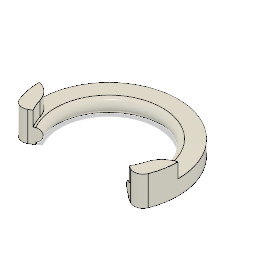
socket_clip (Autodesk Fusion 360 design; units mm, degrees)
Autodesk Fusion 360 part; units mm, degrees
sketch "Sketch6" plane through (0, 0, 0) normal (0, 1, 0) x (1, 0, 0)
  circle A0 centre (0, 0) radius 12
  circle A1 centre (0, 0) radius 9
  dimension "d1" = 24
  dimension "d2" = -3
  constraint coincident A0.centre A1.centre
  measures "d1" diameter of A0
sketch "Sketch3" plane through (0, 0, 0) normal (0, 1, 0) x (1, 0, 0)
  circle A0 centre (0, 0) radius 12.125
  circle A1 centre (0, 0) radius 14.125
  line L0 (0, 0) -> (13.125, 0) construction
  dimension "d18" = 24.25
  dimension "d22" = 2
  constraint coincident A0.centre A1.centre
  constraint horizontal L0
  measures "d18" diameter of A0
sketch "Sketch4" plane through (0, 0, 0) normal (0, 0, 1) x (1, 0, 0)
  line L0 (12.125, 0) -> (10.625, 0)
  line L1 (10.625, 0) -> (10.625, 2.8)
  line L2 (10.625, 2.8) -> (12.125, 2.8)
  line L3 (12.125, 2.8) -> (12.125, 0)
  arc A0 (12.125, 2.8) -> (12.125, 0) centre (12.0283, 1.4) ccw
  line L4 (12.125, 0) -> (15.125, 0)
  line L5 (15.125, 0) -> (15.125, 2.8)
  line L6 (15.125, 2.8) -> (12.125, 2.8)
  line L7 (12.125, 2.8) -> (12.125, 0)
  arc A1 (12.125, 2.8) -> (12.125, 0) centre (11.9125, 1.4) ccw
  dimension "d20" = 1.5
  dimension "d21" = 2.8
  dimension "d23" = 3
  dimension "d24" = 2.8
  dimension "d19" = 1.4033
  constraint horizontal L0
  constraint vertical L1
  constraint horizontal L2
  constraint vertical L3
  constraint tangent L1 A0
  constraint horizontal L4
  constraint vertical L5
  constraint horizontal L6
  constraint vertical L7
  measures "d20" distance of L0.start L0.end
  measures "d21" distance of L0.start L2.end
  measures "d23" distance of L0.start L4.end
  measures "d24" distance of L0.start L2.end
  measures "d19" distance of L1 A0.centre
sweep "Sweep1" add profiles "Sketch4" path "Sketch6" along A1 section 1 contours L1 L2 A0 A1 | L3 A0 L7 | L0 L1 A0 A1 | L3 L4 L5 L6 L7 | L1 A1
sketch "Sketch5" plane through (0, 0, 0) normal (0, -1, 0) x (1, 0, 0)
  circle A0 centre (0, 0) radius 12.125
  circle A1 centre (0, 0) radius 15.125
  line L0 (0, 0) -> (-13.1007, 7.5637)
  line L1 (0, 0) -> (13.0986, 7.5625)
  line L2 (0, 0) -> (0, 17) construction
  circle A2 centre (0, 0) radius 13.125 construction
  line L3 (0, 0) -> (-15.125, 0)
  line L4 (0, 0) -> (15.125, 0)
  dimension "d4" = 60
  dimension "d5" = 60
  dimension "d6" = -2
  dimension "d9" = 90
  dimension "d10" = 17
  dimension "d11" = 90
  constraint coincident A0.centre A1.centre
  constraint coincident A1 L3.end
  constraint coincident A1 L1.end
  constraint coincident A1 L4.end
  constraint vertical L2
  measures "d4" angle of L0 L2
  measures "d5" angle of L1 L2
  measures "d9" angle of L2 L3
  measures "d10" distance of A0.centre L2.end
  measures "d11" angle of L2 L4
extrude "Extrude2" cut sketch "Sketch5" against normal up to surface (2.8 mm away) contours A0 L0 L1 | A0 A1 L0 L1
extrude "Extrude3" add sketch "Sketch5" against normal blind 6 contours A0 A1 L1 L4 | A0 A1 L0 L3
fillet "Fillet1" radius 2 2 edges at (13.0986, 3, 7.5625) (-13.0986, 3, 7.5625)
fillet "Fillet2" radius 5 2 edges at (-12.125, 4.4, 0) (12.125, 4.4, 0)
sketch "Sketch7" plane through (0, 0, 0) normal (0, -1, 0) x (1, 0, 0)
  arc A0 (-11.2338, 6.4859) -> (-14.098, 5.4782) centre (-12.2338, 4.7538) ccw
  arc A1 (-14.098, 5.4782) -> (14.098, 5.4782) centre (0, 0) ccw
  arc A2 (14.098, 5.4782) -> (11.2338, 6.4859) centre (12.2338, 4.7538) ccw
  line L0 (11.2338, 6.4859) -> (10.1325, 5.85)
  line L1 (-10.1325, 5.85) -> (-11.2338, 6.4859)
  arc A3 (-10.1325, 5.85) -> (10.1325, 5.85) centre (0, 0) ccw
extrude "Extrude4" add sketch "Sketch7" along normal blind 0.5
equation "d5 = d4"
equation "d11 = d9"
